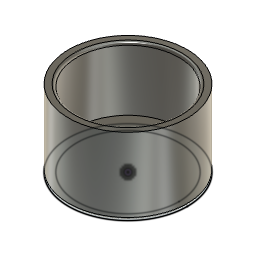
park-tool-pcs-10-foot v1 (Autodesk Fusion 360 design; units mm, degrees)
Autodesk Fusion 360 part; units mm, degrees
sketch "Sketch1" plane through (0, 0, 0) normal (0, 0, 1) x (1, 0, 0)
  circle A0 centre (0, 0) radius 22.5
  circle A1 centre (0, 0) radius 19.35
  dimension "d1" = 45
  dimension "d2" = 38.7
  constraint coincident A0.centre A1.centre
  constraint concentric A0 A1
  measures "d1" diameter of A0
  measures "d2" diameter of A1
extrude "Extrude1" add sketch "Sketch1" along normal blind 5 contours A1
extrude "Extrude2" add sketch "Sketch1" along normal blind 29
fillet "Fillet1" radius 1 1 edges at (-18.0405, 6.9973, 29)
fillet "Fillet2" radius 1 1 edges at (-20.9774, -8.1363, 0)
